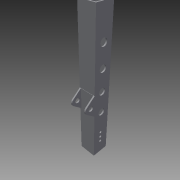
# Autodesk Inventor part: atas 1
Saved by Autodesk Inventor 2014 SP2 (Build 180246200, 246)
## iProperties
Created: 2019-06-24
Part Number: atas 1
Material: Generic
Document SubType Name: Modeling
Designer: USER PC
Density: 1 g/cm^3
Appearance: Default
Author: USER PC
Autodesk Inventor part; units mm, degrees
ref_plane "YZ Plane" through (0, 0, 0) normal (1, 0, 0) x (0, 1, 0)
ref_plane "XZ Plane" through (0, 0, 0) normal (0, 1, 0) x (-1, 0, 0)
ref_plane "XY Plane" through (0, 0, 0) normal (0, 0, 1) x (1, 0, 0)
sketch "Sketch1" plane through (0, 0, 0) normal (0, 0, 1) x (1, 0, 0)
  line L0 (-60, 60) -> (60, 60)
  line L1 (60, 60) -> (60, -60)
  line L2 (60, -60) -> (-60, -60)
  line L3 (-60, -60) -> (-60, 60)
  line L4 (-60, 60) -> (60, -60) construction
  line L5 (60, 60) -> (-60, -60) construction
  point P0 (0, 0)
  dimension "d0" = 120
  dimension "d1" = 120
  constraints: 12 end point, 2 midpoint, 2 parallel, 1 horizontal, 1 perpendicular
  measures "d0" distance of L1.end L2.end
  measures "d1" distance of L0.end L1.end
extrude "Extrusion1" add sketch "Sketch1" along normal blind 1000
sketch "Sketch2" plane through (0, 0, 1000) normal (0, 0, 1) x (1, 0, 0)
  line L0 (-50, 50) -> (50, 50)
  line L1 (50, 50) -> (50, -50)
  line L2 (50, -50) -> (-50, -50)
  line L3 (-50, -50) -> (-50, 50)
  line L4 (-50, 50) -> (50, -50) construction
  line L5 (50, 50) -> (-50, -50) construction
  point P0 (0, 0)
  dimension "d4" = 100
  dimension "d5" = 100
  constraints: 12 end point, 2 midpoint, 2 parallel, 1 horizontal, 1 perpendicular
  measures "d4" distance of L1.end L2.end
  measures "d5" distance of L0.end L1.end
extrude "Extrusion2" cut sketch "Sketch2" against normal blind 1000
sketch "Sketch3" plane through (60, -60, 0) normal (1, 0, 0) x (0, 0, -1)
  line L0 (0, 0) -> (-1000, 0) projected
  line L1 (-1072.8828, 120) -> (-1072.8828, 60)
  line L2 (-1072.8828, 60) -> (45.9524, 60)
  circle A0 centre (-800, 60) radius 25
  line L3 (-1000, 120) -> (-1072.8828, 120)
  line L4 (-1000, 120) -> (-1000, 166.4974)
  line L5 (-800, 60) -> (-800, 166.4974)
  line L6 (-650, 60) -> (-650, 175.0662)
  line L7 (-500, 60) -> (-500, 175.0662)
  circle A1 centre (-650, 60) radius 25
  circle A2 centre (-500, 60) radius 25
  line L8 (-350, 60) -> (-350, 191.0617)
  circle A3 centre (-350, 60) radius 25
  point P0 (0, 60)
  dimension "d9" = 50
  dimension "d10" = 60
  dimension "d12" = 200
  dimension "d13" = 150
  dimension "d14" = 150
  dimension "d15" = 50
  dimension "d16" = 50
  dimension "d17" = 150
  dimension "d18" = 50
  constraints: 16 end point, 5 parallel, 4 centre point, 4 point on line, 3 coincident, 2 perpendicular
  measures "d9" diameter of A0
  measures "d10" distance between parallel lines of L2 L3
  measures "d12" distance between parallel lines of L4 L5
  measures "d13" distance between parallel lines of L6 L5
  measures "d14" distance between parallel lines of L7 L6
  measures "d15" diameter of A1
  measures "d16" diameter of A2
  measures "d17" distance between parallel lines of L8 L7
  measures "d18" diameter of A3
extrude "Extrusion3" cut sketch "Sketch3" against normal blind 1000
sketch "Sketch4" plane through (60, -60, 0) normal (1, 0, 0) x (0, 0, -1)
  line L0 (0, 0) -> (-1000, 0) projected
  line L1 (-1000, -138.0957) -> (-425, -138.0957)
  line L2 (-425, -90) -> (-500, 0)
  line L3 (-425, -90) -> (-350, 0)
  point P0 (0, 60)
  dimension "d21" = 575
  constraints: 6 end point, 1 midpoint, 1 parallel, 1 point on line
  measures "d21" distance of L1.start L1.end
extrude "Extrusion4" add sketch "Sketch4" against normal blind 120
fillet "Fillet1" radius 30 1 edges at (0, -150, 425)
sketch "Sketch5" plane through (60, -60, 0) normal (1, 0, 0) x (0, 0, -1)
  line L0 (-500, 0) -> (-1000, 0) projected
  circle A0 centre (-425, -30) radius 17.5
  line L1 (-425, -6.2892) -> (-425, -12.5)
  point P0 (0, 60)
  constraints: 2 end point, 1 perpendicular, 1 vertical alignment, 2 other
extrude "Extrusion5" cut sketch "Sketch5" against normal blind 120
sketch "Sketch11" plane through (0, 0, 0) normal (1, 0, 0) x (0, 1, 0)
  line L0 (0, 0) -> (-191.3129, 0)
  line L1 (-191.3129, 0) -> (-191.3129, 1000)
  line L2 (-340.1694, 1000) -> (-340.1694, 500)
  line L3 (-340.1694, 500) -> (94.4413, 500)
  line L4 (-60.9651, 500) -> (-60.9651, 425)
  line L5 (-150.9651, 425) -> (-60.9651, 500)
  line L6 (-60.9651, 425) -> (-60.9651, 350)
  line L7 (-60.9651, 350) -> (-150.9651, 425)
  dimension "d33" = 1000
  dimension "d35" = 500
  constraints: 16 end point, 3 perpendicular, 1 horizontal, 1 parallel, 1 point on line
  measures "d33" distance of L0.end L1.end
  measures "d35" distance of L2.start L2.end
extrude "Extrusion6" cut sketch "Sketch11" along normal mid plane 100
sketch "Sketch12" plane through (60, -60, 0) normal (1, 0, 0) x (0, 0, -1)
  circle A0 centre (-100, 60) radius 10
  circle A1 centre (-140, 60) radius 10
  circle A2 centre (-180, 60) radius 10
  point P0 (0, 60)
  dimension "d41" = 20
  dimension "d42" = 20
  dimension "d43" = 20
  dimension "d44" = 40
  dimension "d45" = 40
  dimension "d46" = 100
  constraints: 3 centre point
  measures "d41" diameter of A0
  measures "d42" diameter of A1
  measures "d43" diameter of A2
  measures "d44" distance of A1.centre A2.centre
  measures "d45" distance of A0.centre A1.centre
  measures "d46" distance of point (0, 60) A0.centre
extrude "Extrusion7" cut sketch "Sketch12" against normal blind 599.25
body "Solid1"
